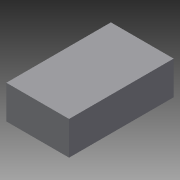
# Autodesk Inventor part: PSU
Saved by Autodesk Inventor 2015 (Build 190159000, 159)
## iProperties
Created: 2015-06-19
Part Number: PSU
Material: Generic
Document SubType Name: Modeling
Designer: smkilani
Density: 1 g/cm^3
Appearance: Default
Author: smkilani
Autodesk Inventor part; units mm, degrees
ref_plane "YZ Plane" through (0, 0, 0) normal (1, 0, 0) x (0, 1, 0)
ref_plane "XZ Plane" through (0, 0, 0) normal (0, 1, 0) x (-1, 0, 0)
ref_plane "XY Plane" through (0, 0, 0) normal (0, 0, 1) x (1, 0, 0)
sketch "Sketch1" plane through (0, 0, 0) normal (0, 0, 1) x (1, 0, 0)
  line L0 (57.15, 30.5) -> (-57.15, 30.5)
  line L1 (-57.15, 30.5) -> (-57.15, -30.5)
  line L2 (-57.15, -30.5) -> (57.15, -30.5)
  line L3 (57.15, -30.5) -> (57.15, 30.5)
  line L4 (57.15, 30.5) -> (-57.15, -30.5) construction
  line L5 (-57.15, 30.5) -> (57.15, -30.5) construction
  point P0 (0, 0)
  dimension "d0" = 114.3
  dimension "d1" = 61
  constraints: 12 end point, 2 midpoint, 2 parallel, 1 horizontal, 1 perpendicular
  measures "d0" distance of L2.end L1.end
  measures "d1" distance of L1.end L0.end
extrude "Extrusion1" add sketch "Sketch1" along normal blind 190.5
body "Solid1"
